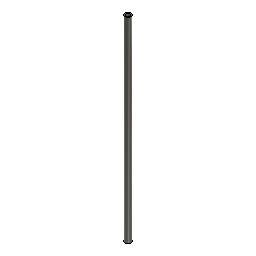
2차 예선 모델링_ADW (Autodesk Fusion 360 archive; units mm, degrees)
design "Aluminum 4mm 6mm bar"
Autodesk Fusion 360 part; units mm, degrees
sketch "Aluminum 4mm-6mm" plane through (0, 0, 0) normal (0, 0, 1) x (1, 0, 0)
  circle A0 centre (0, 0) radius 2
  circle A1 centre (0, 0) radius 3
  dimension "d1" = 4
  dimension "d2" = 6
  constraint coincident A0.centre A1.centre
  measures "d1" diameter of A0
  measures "d2" diameter of A1
extrude "Extrude1" add sketch "Aluminum 4mm-6mm" along normal blind 190 makes body 1
copy_body "Body->Comp1" bodies 1 removing the originals makes body 2 in component "190mm aluminum 4-6 bar"
extrude "Extrude2" add sketch "Aluminum 4mm-6mm" along normal blind 250 separate body makes body 3
copy_body "Body->Comp2" bodies 3 removing the originals makes body 4 in component "250mm aluminum 4-6 bar"
extrude "Extrude3" add sketch "Aluminum 4mm-6mm" along normal blind 120 separate body makes body 5
copy_body "Body->Comp3" bodies 5 removing the originals makes body 6 in component "120mm aluminum 4-6 bar"
extrude "Extrude4" add sketch "Aluminum 4mm-6mm" along normal blind 222 separate body makes body 7
copy_body "Body->Comp4" bodies 7 removing the originals makes body 8 in component "220mm aluminum 4-6 bar"
extrude "Extrude5" add sketch "Aluminum 4mm-6mm" along normal blind 30 separate body makes body 9
copy_body "Body->Comp5" bodies 9 removing the originals makes body 10 in component "30mm aluminum 4-6 bar"
component "190mm aluminum 4-6 bar" placed x (1, 0, 0) y (0, 1, 0) z (0, 0, 1) at (0, 0, 0)
component "250mm aluminum 4-6 bar" placed x (1, 0, 0) y (0, 1, 0) z (0, 0, 1) at (0, 0, 0)
component "120mm aluminum 4-6 bar" placed x (1, 0, 0) y (0, 1, 0) z (0, 0, 1) at (0, 0, 0)
component "220mm aluminum 4-6 bar" placed x (1, 0, 0) y (0, 1, 0) z (0, 0, 1) at (0, 0, 0)
component "30mm aluminum 4-6 bar" placed x (1, 0, 0) y (0, 1, 0) z (0, 0, 1) at (0, 0, 0)
equation "d13 = 180 mm + ( ( 5 + 5 + 3 + 8 ) * 2 ) * 1 mm"

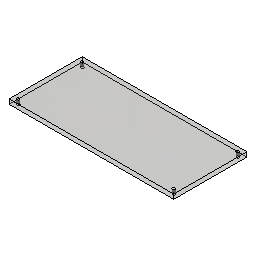
design "Simple Flat Bucket"
Autodesk Fusion 360 part; units mm, degrees
sketch "Sketch1" plane through (0, 0, 0) normal (0, 0, 1) x (1, 0, 0)
  line L0 (90, -40) -> (-90, -40)
  line L1 (-90, -40) -> (-90, 40)
  line L2 (-90, 40) -> (90, 40)
  line L3 (90, 40) -> (90, -40)
  line L4 (90, -40) -> (-90, 40) construction
  line L5 (-90, -40) -> (90, 40) construction
  line L6 (-85, -35) -> (85, 35) construction
  line L7 (85, -35) -> (-85, 35) construction
  circle A0 centre (-85, 35) radius 1.5
  circle A1 centre (-85, -35) radius 1.5
  circle A2 centre (85, 35) radius 1.5
  circle A3 centre (85, -35) radius 1.5
  dimension "d1" = 180
  dimension "d2" = 80
  dimension "d3" = 170
  dimension "d4" = 70
  dimension "d5" = 3
  dimension "d6" = 3
  dimension "d7" = 3
  dimension "d8" = 3
  constraint horizontal L0
  constraint perpendicular L0 L1
  constraint parallel L0 L2
  constraint parallel L1 L3
  constraint coincident L4 origin
  constraint coincident L5 origin
  constraint coincident L6 origin
  constraint coincident L7 origin
  constraint coincident L7.end A0.centre
  constraint coincident L6.start A1.centre
  constraint coincident L6.end A2.centre
  constraint coincident L7.start A3.centre
  measures "d1" distance of L1.end L2.end
  measures "d2" distance of L0.end L1.end
  measures "d3" distance of L6.end L7.end
  measures "d4" distance of L7.start L6.end
  measures "d5" diameter of A0
  measures "d6" diameter of A1
  measures "d7" diameter of A2
  measures "d8" diameter of A3
extrude "Extrude1" add sketch "Sketch1" along normal blind 5 makes body 1
copy_body "Body->Comp1" bodies 1 removing the originals makes body 2 in component "Simple flat bucket"
component "Simple flat bucket" placed x (1, 0, 0) y (0, 1, 0) z (0, 0, 1) at (0, 0, 0)

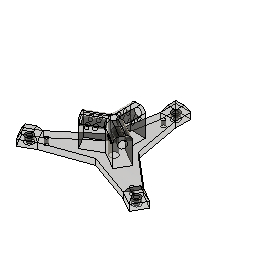
design "90mm_Center Piece 3 Cap"
Autodesk Fusion 360 part; units mm, degrees
sketch "스케치1" plane through (0, 0, 0) normal (0, 0, 1) x (1, 0, 0)
  circle A0 centre (0, 0) radius 45
  circle A1 centre (0, 0) radius 3.25
  line L0 (0, 0) -> (0, 45)
  line L1 (0, 3.25) -> (0, 7.25)
  line L2 (0, 45) -> (0, 41)
  circle A2 centre (0, 7.25) radius 1.5
  circle A3 centre (0, 41) radius 1.5
  circle A4 centre (-6.278684, -3.625) radius 1.5
  circle A5 centre (-35.507042, -20.5) radius 1.5
  circle A6 centre (6.278684, -3.625) radius 1.5
  circle A7 centre (35.507042, -20.5) radius 1.5
  line L3 (0, 45) -> (0, 57.5)
  line L4 (0, 57.5) -> (6.25, 57.5)
  line L5 (6.25, 57.5) -> (6.25, 44.563859)
  line L6 (0, 57.5) -> (-6.25, 57.5)
  line L7 (-6.25, 57.5) -> (-6.25, 44.563859)
  circle A8 centre (0, 51.25) radius 3.25
  circle A9 centre (0, 51.25) radius 1.75
  line L8 (-46.671461, -34.162659) -> (-35.468434, -27.694588)
  circle A10 centre (-44.383802, -25.625) radius 3.25
  circle A11 centre (-44.383802, -25.625) radius 1.75
  line L9 (-49.796461, -28.75) -> (-46.671461, -34.162659)
  line L10 (-49.796461, -28.75) -> (-52.921461, -23.337341)
  line L11 (-52.921461, -23.337341) -> (-41.718434, -16.869271)
  line L12 (52.921461, -23.337341) -> (41.718434, -16.869271)
  circle A12 centre (44.383802, -25.625) radius 3.25
  circle A13 centre (44.383802, -25.625) radius 1.75
  line L13 (49.796461, -28.75) -> (52.921461, -23.337341)
  line L14 (49.796461, -28.75) -> (46.671461, -34.162659)
  line L15 (46.671461, -34.162659) -> (35.468434, -27.694588)
  spline S0 degree 5 poles (35.468434, -27.694588) (34.819906, -27.317495) (33.509104, -26.546566) (31.501491, -25.340032) (28.579456, -23.675318) (23.424733, -21.747786) (16.754594, -20.597941) (9.434581, -20.121161) (3.346407, -20.006491) (0, -20) knots 0 0 0 0 0 0 0.2 0.4 0.6 0.8 1 1 1 1 1 1
  line L16 (8.439143, -20.016369) -> (-8.439143, -19.983631)
  line L17 (37.082946, -28.633365) -> (33.853922, -26.755812)
  line L18 (0, 0) -> (-0.087287, -44.999915)
  spline S1 degree 5 poles (-35.575605, -27.556783) (-34.92562, -27.182208) (-33.611836, -26.416371) (-31.599558, -25.217634) (-28.671087, -23.564268) (-23.508925, -21.656748) (-16.834376, -20.532788) (-9.512568, -20.084409) (-3.423995, -19.993358) (-0.077588, -19.99985) knots 0 0 0 0 0 0 0.2 0.4 0.6 0.8 1 1 1 1 1 1
  line L19 (-37.193747, -28.489289) -> (-33.957463, -26.624277)
  line L20 (-8.516731, -19.98348) -> (8.361555, -20.016219)
  spline S2 degree 5 poles (6.25, 44.563859) (6.247691, 43.813671) (6.235449, 42.293018) (6.194366, 39.951107) (6.213699, 36.588193) (7.121768, 31.160307) (9.461043, 24.808875) (12.708146, 18.231167) (15.652926, 12.901319) (17.320508, 10) knots 0 0 0 0 0 0 0.2 0.4 0.6 0.8 1 1 1 1 1 1
  spline S3 degree 5 poles (41.652677, -17.030986) (41.003293, -16.65537) (39.683167, -15.900518) (37.638891, -14.757203) (34.742798, -13.047755) (30.509756, -9.530952) (26.199104, -4.312603) (22.149892, 1.804079) (19.026754, 7.031413) (17.359172, 9.932731) knots 0 0 0 0 0 0 0.2 0.4 0.6 0.8 1 1 1 1 1 1
  spline S4 degree 5 poles (-41.718434, -16.869271) (-41.067597, -16.496176) (-39.744553, -15.746452) (-37.695857, -14.611075) (-34.793154, -12.912876) (-30.546501, -9.412521) (-26.215638, -4.210934) (-22.142727, 1.889994) (-18.999333, 7.105172) (-17.320508, 10) knots 0 0 0 0 0 0 0.2 0.4 0.6 0.8 1 1 1 1 1 1
  spline S5 degree 5 poles (-6.077072, 44.58777) (-6.077673, 43.837578) (-6.07133, 42.31689) (-6.039333, 39.974837) (-6.071712, 36.612024) (-7.000831, 31.1877) (-9.364728, 24.845392) (-12.637324, 18.28033) (-15.602759, 12.961946) (-17.281584, 10.067118) knots 0 0 0 0 0 0 0.2 0.4 0.6 0.8 1 1 1 1 1 1
  point P0 (0, -20)
  dimension "d1" = 90
  dimension "d2" = 6.5
  dimension "d3" = 4
  dimension "d4" = 4
  dimension "d5" = 3
  dimension "d6" = 3
  dimension "d8" = 360
  dimension "d21" = 12.5
  dimension "d22" = 6.25
  dimension "d23" = 6.5
  dimension "d24" = 3.5
  dimension "d33" = 360
  constraint coincident A0.centre A1.centre
  constraint coincident A0 L0.end
  constraint vertical L0
  constraint coincident A1 L1.start
  constraint coincident L0 L1.start
  constraint parallel L0 L1
  constraint parallel L0 L2
  constraint coincident L1.end A2.centre
  constraint coincident L2.end A3.centre
  constraint parallel L2 L3
  constraint perpendicular L3 L4
  constraint perpendicular L4 L5
  constraint symmetric L4.start L3 L6.start
  constraint symmetric L3 L4.end L6.end
  constraint midpoint L3 A8.centre
  constraint concentric A8 A9
  constraint coincident P0 S0.end
  constraint midpoint P0 L16
  constraint perpendicular L16 L18
  measures "d1" diameter of A0
  measures "d2" diameter of A1
  measures "d3" distance of L1.start L1.end
  measures "d4" distance of L0.end L2.end
  measures "d5" diameter of A2
  measures "d6" diameter of A3
  measures "d21" distance of L0.end L3.end
  measures "d22" distance of L3.end L4.end
  measures "d23" diameter of A8
  measures "d24" diameter of A9
extrude "돌출4" add sketch "스케치1" along normal blind 5 contours A0 A1 L0 L1 L2 A2 A3 S0 L16 L18 L20 | A0 L3 L4 L5 A8 | A0 L12 L13 L14 L15 | A0 A1 L0 L1 L2 A2 A3 L16 L18 S1 L20 | A0 L3 L6 L7 A8 | A0 S0 L16 L18 L20 | A0 L16 L18 S1 L20 | A0 L8 L9 L10 L11 | L0 L1 A2 | L0 L1 A2 | A4 | A6 picked at (6.734071, 29.745011) picked at (5.25, 51.10462) picked at (41.632899, -30.098943) picked at (-29.096092, -9.179545) picked at (-5.246971, 51.023662) picked at (5.130061, -28.288576) picked at (-5.231524, -28.269552) picked at (-46.882899, -21.005676) picked at (0.934562, 6.901426) picked at (-0.074521, 6.255585) picked at (-6.318535, -3.159563) picked at (6.238834, -3.159563) makes body 1
extrude "돌출5" add sketch "스케치1" along normal blind 5 draft -30 from surface at 5 contours A0 L3 L4 L5 A8 | A0 L12 L13 L14 L15 | A0 L3 L6 L7 A8 | L3 A8 A9 | L3 A8 A9 | L3 A9 | L3 A9 | A0 L8 L9 L10 L11 | A10 | A11 | A12 | A13 picked at (5.25, 51.10462) picked at (41.632899, -30.098943) picked at (-5.246971, 51.023662) picked at (-0.248404, 48.518615) picked at (2.733036, 51.012809) picked at (-0.753643, 50.736175) picked at (0.998553, 50.82811) picked at (-46.882899, -21.005676) picked at (-41.652417, -25.873404) picked at (-44.941219, -25.453059) picked at (47.115187, -25.873404) picked at (43.826384, -25.453059) bodies 1
extrude "돌출6" add sketch "스케치1" along normal blind 5 contours L3 A9 | L3 A9 | A11 | A13 picked at (-0.753643, 50.736175) picked at (0.998553, 50.82811) picked at (-44.941219, -25.453059) picked at (43.826384, -25.453059) bodies 1
copy_body "본체->구성요소2" bodies 1 removing the originals makes body 2 in component "90mm_3flapcap"
extrude "Extrude1" add 1 faces at (-27.563056, -7.985641, 5) along direction (0, 0, 1) blind 5 on bodies 2 bodies 2 in component "90mm_3flapcap"
sketch "Sketch6" plane through (0, 0, 10) normal (0, 0, 1) x (-1, 0, 0)
  line L0 (0, 0) -> (-6, 0)
  line L1 (-6, 0) -> (-6, -20)
  circle A0 centre (0, 0) radius 3.25
  line L2 (0, -3.25) -> (0, 0)
  line L3 (6, 0) -> (6, -20)
  line L4 (0, 0) -> (6, 0)
  line L5 (-6, -20) -> (6, -20)
  dimension "d36" = 6
  dimension "d37" = 20
  constraint coincident L0.start A0.centre
  constraint horizontal L0
  constraint perpendicular L0 L1
  constraint coincident A0 L2.start
  constraint perpendicular L0 L2
  constraint symmetric L0.start L2 A0.centre
  constraint symmetric L0.end L2 L3.start
  constraint symmetric L1.end L2 L3.end
  measures "d36" distance of L0.start L0.end
  measures "d37" distance of L0.end L1.end
extrude "Extrude2" add sketch "Sketch6" along normal blind 5 separate body contours L0 L1 A0 L3 L4 L5 picked at (0, -14.416667) makes body 3 in component "90mm_3flapcap"
extrude "Extrude3" add 1 faces at (0, 14.416667, 15) along direction (0, 0, 1) blind 12 on bodies 3 bodies 3 2 in component "90mm_3flapcap"
sketch "Sketch7" plane through (0, 20, 0) normal (0, 1, 0) x (-1, 0, 0)
  line L0 (-3.25, 27) -> (3.25, 27)
  line L1 (0, 27) -> (0, 24)
  line L2 (0, 24) -> (0, 21)
  circle A0 centre (0, 21) radius 3.05
  dimension "d42" = 3
  dimension "d43" = 3
  dimension "d44" = 6.1
  constraint midpoint L0 L1.start
  constraint perpendicular L0 L1
  constraint parallel L1 L2
  constraint coincident L2.end A0.centre
  measures "d42" distance of L1.start L1.end
  measures "d43" distance of L1.end L2.end
  measures "d44" diameter of A0
extrude "Extrude4" cut sketch "Sketch7" against normal blind 15 contours A0 picked at (-0.907334, 21.904758) bodies 2 3 in component "90mm_3flapcap"
fillet "Fillet1" radius 4 2 edges at (-6, 10, 27) (6, 10, 27) on bodies 3 in component "90mm_3flapcap"
sketch "Sketch8" plane through (-6, 0, 0) normal (-1, 0, 0) x (0, -1, 0)
  line L0 (-20, 10) -> (-20, 23)
  line L1 (-20, 21) -> (-5, 21)
  line L2 (-5, 21) -> (-10, 21)
  line L3 (-20, 21) -> (-15, 21)
  circle A0 centre (-15, 21) radius 1.5
  circle A1 centre (-10, 21) radius 1.5
  point P0 (-20, 21)
  point P1 (-5, 21)
  dimension "d49" = 5
  dimension "d50" = 5
  dimension "d51" = 3
  dimension "d52" = 3
  constraint coincident P0 L1.start
  constraint coincident P1 L1.end
  constraint perpendicular L0 L2
  constraint perpendicular L0 L3
  constraint coincident L3.end A0.centre
  constraint coincident L2.end A1.centre
  measures "d49" distance of P1 L2.end
  measures "d50" distance of P0 L3.end
  measures "d51" diameter of A0
  measures "d52" diameter of A1
extrude "Extrude5" cut sketch "Sketch8" against normal blind 13.303 contours L1 L3 A0 | L1 L3 A0 | L1 L2 A1 | L1 L2 A1 picked at (-15.994415, 21.074521) picked at (-14.005585, 20.925479) picked at (-10.863604, 21.498602) picked at (-10.994415, 20.925479) bodies 3 in component "90mm_3flapcap"
pattern_circular "C-Pattern1" count 3 over 360 about axis through (0, 0, 1.75) along (0, 0, 1) of bodies 3 makes body 4 at (-8.922965, -7.912292, 19.106128) makes body 5 at (11.313728, -3.771368, 19.106128) in component "90mm_3flapcap"
combine "Combine1" operation add target body 2 tool bodies 4 5 3 in component "90mm_3flapcap"
extrude "Extrude6" cut 1 faces at (-22.255559, 11.640654, 10) along direction (0, 0, -1) blind 5 on bodies 2 bodies 2 in component "90mm_3flapcap"
sketch "Sketch9" plane through (0, 0, 5) normal (0, 0, 1) x (-1, 0, 0)
  circle A0 centre (0, 0) radius 45
  line L0 (-35.468434, 27.694588) -> (-46.671461, 34.162659)
  line L1 (-41.069947, 30.928623) -> (-26.727174, 22.647819)
  arc A1 (35.468434, 27.694588) -> (-35.468434, 27.694588) centre (0, 0) ccw
  line L2 (0, 0) -> (0, 45)
  line L3 (-35.468434, 27.694588) -> (0, 15)
  line L4 (35.468434, 27.694588) -> (0, 15)
  line L5 (-6.25, -44.563859) -> (-12.990381, -7.5)
  line L6 (-41.718434, 16.869271) -> (-12.990381, -7.5)
  line L7 (41.718434, 16.869271) -> (12.990381, -7.5)
  line L8 (6.25, -44.563859) -> (12.990381, -7.5)
  line L9 (0, 0) -> (0, 15)
  dimension "d60" = 360
  dimension "d63" = 15
  constraint coincident A0.centre A1.centre
  constraint parallel L0 L1
  constraint midpoint A1 L2.end
  constraint coincident L2 L3.end
  constraint symmetric L2 L3.end L4.end
  constraint parallel L2 L9
  constraint coincident L3.end L4.end
  measures "d63" distance of A0.centre L3.end
extrude "Extrude7" cut sketch "Sketch9" against normal blind 25 contours A0 L7 L8 | A0 A1 L2 L4 | A0 L5 L6 | A0 A1 L2 L3 picked at (30.575697, -16.872457) picked at (1.939961, 34.874023) picked at (-30.247561, -17.463438) picked at (-1.939961, 34.874023) bodies 2 in component "90mm_3flapcap"
component "90mm_3flapcap" placed x (1, 0, 0) y (0, 1, 0) z (0, 0, 1) at (0, 0, 0)
equation "d21 = 6.5 mm + ( 3 * 2 ) * 1 mm"
equation "d22 = ( 6.5 / 2 ) * 1 mm + 3 mm"

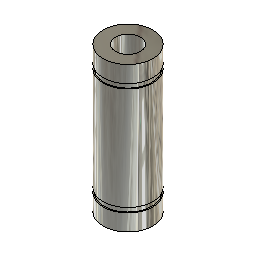
design "LM6L"
Autodesk Fusion 360 part; units mm, degrees
sketch "Sketch1" plane through (0, 0, 0) normal (0, 0, 1) x (1, 0, 0)
  circle A0 centre (0, 0) radius 6
  circle A1 centre (0, 0) radius 3
  dimension "d1" = 12
  dimension "d2" = 6
  constraint coincident A0.centre A1.centre
  constraint concentric A0 A1
  measures "d1" diameter of A0
  measures "d2" diameter of A1
extrude "Extrude1" add sketch "Sketch1" along normal blind 35 makes body 1
sketch "Sketch2" plane through (0, 0, 35) normal (0, 0, 1) x (-1, 0, 0)
  circle A0 centre (0, 0) radius 5.75
  circle A1 centre (0, 0) radius 6
  dimension "d5" = 11.5
  dimension "d6" = 12
  constraint coincident A0.centre A1.centre
  measures "d5" diameter of A0
  measures "d6" diameter of A1
extrude "Extrude2" add sketch "Sketch2" against normal blind 1.1 from surface at -4 separate body makes body 2
ref_plane "WorkPlane1" through (0, 0, 17.5) normal (0, 0, -1) x (-1, 0, 0)
mirror "Mirror1" about plane through (0, 0, 17.5) normal (0, 0, -1) of bodies 2 makes body 3
combine "Combine1" operation cut target body 1 tool bodies 2 3
copy_body "Body->Comp1" bodies 1 removing the originals makes body 4 in component "LM6L"
component "LM6L" placed x (1, 0, 0) y (0, 1, 0) z (0, 0, 1) at (0, 0, 0)
equation "d7 = ( -( 35 - 27 ) / 2 ) * 1 mm"
named bodies: "LM6L"

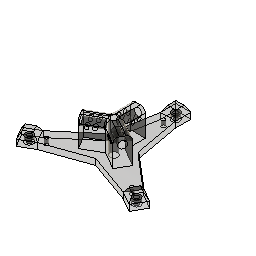
design "90mm_Center Piece 3 Cap"
Autodesk Fusion 360 part; units mm, degrees
sketch "스케치1" plane through (0, 0, 0) normal (0, 0, 1) x (1, 0, 0)
  circle A0 centre (0, 0) radius 45
  circle A1 centre (0, 0) radius 3.25
  line L0 (0, 0) -> (0, 45)
  line L1 (0, 3.25) -> (0, 7.25)
  line L2 (0, 45) -> (0, 41)
  circle A2 centre (0, 7.25) radius 1.5
  circle A3 centre (0, 41) radius 1.5
  circle A4 centre (-6.278684, -3.625) radius 1.5
  circle A5 centre (-35.507042, -20.5) radius 1.5
  circle A6 centre (6.278684, -3.625) radius 1.5
  circle A7 centre (35.507042, -20.5) radius 1.5
  line L3 (0, 45) -> (0, 57.5)
  line L4 (0, 57.5) -> (6.25, 57.5)
  line L5 (6.25, 57.5) -> (6.25, 44.563859)
  line L6 (0, 57.5) -> (-6.25, 57.5)
  line L7 (-6.25, 57.5) -> (-6.25, 44.563859)
  circle A8 centre (0, 51.25) radius 3.25
  circle A9 centre (0, 51.25) radius 1.75
  line L8 (-46.671461, -34.162659) -> (-35.468434, -27.694588)
  circle A10 centre (-44.383802, -25.625) radius 3.25
  circle A11 centre (-44.383802, -25.625) radius 1.75
  line L9 (-49.796461, -28.75) -> (-46.671461, -34.162659)
  line L10 (-49.796461, -28.75) -> (-52.921461, -23.337341)
  line L11 (-52.921461, -23.337341) -> (-41.718434, -16.869271)
  line L12 (52.921461, -23.337341) -> (41.718434, -16.869271)
  circle A12 centre (44.383802, -25.625) radius 3.25
  circle A13 centre (44.383802, -25.625) radius 1.75
  line L13 (49.796461, -28.75) -> (52.921461, -23.337341)
  line L14 (49.796461, -28.75) -> (46.671461, -34.162659)
  line L15 (46.671461, -34.162659) -> (35.468434, -27.694588)
  spline S0 degree 5 poles (35.468434, -27.694588) (34.819906, -27.317495) (33.509104, -26.546566) (31.501491, -25.340032) (28.579456, -23.675318) (23.424733, -21.747786) (16.754594, -20.597941) (9.434581, -20.121161) (3.346407, -20.006491) (0, -20) knots 0 0 0 0 0 0 0.2 0.4 0.6 0.8 1 1 1 1 1 1
  line L16 (8.439143, -20.016369) -> (-8.439143, -19.983631)
  line L17 (37.082946, -28.633365) -> (33.853922, -26.755812)
  line L18 (0, 0) -> (-0.087287, -44.999915)
  spline S1 degree 5 poles (-35.575605, -27.556783) (-34.92562, -27.182208) (-33.611836, -26.416371) (-31.599558, -25.217634) (-28.671087, -23.564268) (-23.508925, -21.656748) (-16.834376, -20.532788) (-9.512568, -20.084409) (-3.423995, -19.993358) (-0.077588, -19.99985) knots 0 0 0 0 0 0 0.2 0.4 0.6 0.8 1 1 1 1 1 1
  line L19 (-37.193747, -28.489289) -> (-33.957463, -26.624277)
  line L20 (-8.516731, -19.98348) -> (8.361555, -20.016219)
  spline S2 degree 5 poles (6.25, 44.563859) (6.247691, 43.813671) (6.235449, 42.293018) (6.194366, 39.951107) (6.213699, 36.588193) (7.121768, 31.160307) (9.461043, 24.808875) (12.708146, 18.231167) (15.652926, 12.901319) (17.320508, 10) knots 0 0 0 0 0 0 0.2 0.4 0.6 0.8 1 1 1 1 1 1
  spline S3 degree 5 poles (41.652677, -17.030986) (41.003293, -16.65537) (39.683167, -15.900518) (37.638891, -14.757203) (34.742798, -13.047755) (30.509756, -9.530952) (26.199104, -4.312603) (22.149892, 1.804079) (19.026754, 7.031413) (17.359172, 9.932731) knots 0 0 0 0 0 0 0.2 0.4 0.6 0.8 1 1 1 1 1 1
  spline S4 degree 5 poles (-41.718434, -16.869271) (-41.067597, -16.496176) (-39.744553, -15.746452) (-37.695857, -14.611075) (-34.793154, -12.912876) (-30.546501, -9.412521) (-26.215638, -4.210934) (-22.142727, 1.889994) (-18.999333, 7.105172) (-17.320508, 10) knots 0 0 0 0 0 0 0.2 0.4 0.6 0.8 1 1 1 1 1 1
  spline S5 degree 5 poles (-6.077072, 44.58777) (-6.077673, 43.837578) (-6.07133, 42.31689) (-6.039333, 39.974837) (-6.071712, 36.612024) (-7.000831, 31.1877) (-9.364728, 24.845392) (-12.637324, 18.28033) (-15.602759, 12.961946) (-17.281584, 10.067118) knots 0 0 0 0 0 0 0.2 0.4 0.6 0.8 1 1 1 1 1 1
  point P0 (0, -20)
  dimension "d1" = 90
  dimension "d2" = 6.5
  dimension "d3" = 4
  dimension "d4" = 4
  dimension "d5" = 3
  dimension "d6" = 3
  dimension "d8" = 360
  dimension "d21" = 12.5
  dimension "d22" = 6.25
  dimension "d23" = 6.5
  dimension "d24" = 3.5
  dimension "d33" = 360
  constraint coincident A0.centre A1.centre
  constraint coincident A0 L0.end
  constraint vertical L0
  constraint coincident A1 L1.start
  constraint coincident L0 L1.start
  constraint parallel L0 L1
  constraint parallel L0 L2
  constraint coincident L1.end A2.centre
  constraint coincident L2.end A3.centre
  constraint parallel L2 L3
  constraint perpendicular L3 L4
  constraint perpendicular L4 L5
  constraint symmetric L4.start L3 L6.start
  constraint symmetric L3 L4.end L6.end
  constraint midpoint L3 A8.centre
  constraint concentric A8 A9
  constraint coincident P0 S0.end
  constraint midpoint P0 L16
  constraint perpendicular L16 L18
  measures "d1" diameter of A0
  measures "d2" diameter of A1
  measures "d3" distance of L1.start L1.end
  measures "d4" distance of L0.end L2.end
  measures "d5" diameter of A2
  measures "d6" diameter of A3
  measures "d21" distance of L0.end L3.end
  measures "d22" distance of L3.end L4.end
  measures "d23" diameter of A8
  measures "d24" diameter of A9
extrude "돌출4" add sketch "스케치1" along normal blind 5 contours A0 A1 L0 L1 L2 A2 A3 S0 L16 L18 L20 | A0 L3 L4 L5 A8 | A0 L12 L13 L14 L15 | A0 A1 L0 L1 L2 A2 A3 L16 L18 S1 L20 | A0 L3 L6 L7 A8 | A0 S0 L16 L18 L20 | A0 L16 L18 S1 L20 | A0 L8 L9 L10 L11 | L0 L1 A2 | L0 L1 A2 | A4 | A6 picked at (6.734071, 29.745011) picked at (5.25, 51.10462) picked at (41.632899, -30.098943) picked at (-29.096092, -9.179545) picked at (-5.246971, 51.023662) picked at (5.130061, -28.288576) picked at (-5.231524, -28.269552) picked at (-46.882899, -21.005676) picked at (0.934562, 6.901426) picked at (-0.074521, 6.255585) picked at (-6.318535, -3.159563) picked at (6.238834, -3.159563) makes body 1
extrude "돌출5" add sketch "스케치1" along normal blind 5 draft -30 from surface at 5 contours A0 L3 L4 L5 A8 | A0 L12 L13 L14 L15 | A0 L3 L6 L7 A8 | L3 A8 A9 | L3 A8 A9 | L3 A9 | L3 A9 | A0 L8 L9 L10 L11 | A10 | A11 | A12 | A13 picked at (5.25, 51.10462) picked at (41.632899, -30.098943) picked at (-5.246971, 51.023662) picked at (-0.248404, 48.518615) picked at (2.733036, 51.012809) picked at (-0.753643, 50.736175) picked at (0.998553, 50.82811) picked at (-46.882899, -21.005676) picked at (-41.652417, -25.873404) picked at (-44.941219, -25.453059) picked at (47.115187, -25.873404) picked at (43.826384, -25.453059) bodies 1
extrude "돌출6" add sketch "스케치1" along normal blind 5 contours L3 A9 | L3 A9 | A11 | A13 picked at (-0.753643, 50.736175) picked at (0.998553, 50.82811) picked at (-44.941219, -25.453059) picked at (43.826384, -25.453059) bodies 1
copy_body "본체->구성요소2" bodies 1 removing the originals makes body 2 in component "90mm_3flapcap"
extrude "Extrude1" add 1 faces at (-27.563056, -7.985641, 5) along direction (0, 0, 1) blind 5 on bodies 2 bodies 2 in component "90mm_3flapcap"
sketch "Sketch6" plane through (0, 0, 10) normal (0, 0, 1) x (-1, 0, 0)
  line L0 (0, 0) -> (-6, 0)
  line L1 (-6, 0) -> (-6, -20)
  circle A0 centre (0, 0) radius 3.25
  line L2 (0, -3.25) -> (0, 0)
  line L3 (6, 0) -> (6, -20)
  line L4 (0, 0) -> (6, 0)
  line L5 (-6, -20) -> (6, -20)
  dimension "d36" = 6
  dimension "d37" = 20
  constraint coincident L0.start A0.centre
  constraint horizontal L0
  constraint perpendicular L0 L1
  constraint coincident A0 L2.start
  constraint perpendicular L0 L2
  constraint symmetric L0.start L2 A0.centre
  constraint symmetric L0.end L2 L3.start
  constraint symmetric L1.end L2 L3.end
  measures "d36" distance of L0.start L0.end
  measures "d37" distance of L0.end L1.end
extrude "Extrude2" add sketch "Sketch6" along normal blind 5 separate body contours L0 L1 A0 L3 L4 L5 picked at (0, -14.416667) makes body 3 in component "90mm_3flapcap"
extrude "Extrude3" add 1 faces at (0, 14.416667, 15) along direction (0, 0, 1) blind 12 on bodies 3 bodies 3 2 in component "90mm_3flapcap"
sketch "Sketch7" plane through (0, 20, 0) normal (0, 1, 0) x (-1, 0, 0)
  line L0 (-3.25, 27) -> (3.25, 27)
  line L1 (0, 27) -> (0, 24)
  line L2 (0, 24) -> (0, 21)
  circle A0 centre (0, 21) radius 3.05
  dimension "d42" = 3
  dimension "d43" = 3
  dimension "d44" = 6.1
  constraint midpoint L0 L1.start
  constraint perpendicular L0 L1
  constraint parallel L1 L2
  constraint coincident L2.end A0.centre
  measures "d42" distance of L1.start L1.end
  measures "d43" distance of L1.end L2.end
  measures "d44" diameter of A0
extrude "Extrude4" cut sketch "Sketch7" against normal blind 15 contours A0 picked at (-0.907334, 21.904758) bodies 2 3 in component "90mm_3flapcap"
fillet "Fillet1" radius 4 2 edges at (-6, 10, 27) (6, 10, 27) on bodies 3 in component "90mm_3flapcap"
sketch "Sketch8" plane through (-6, 0, 0) normal (-1, 0, 0) x (0, -1, 0)
  line L0 (-20, 10) -> (-20, 23)
  line L1 (-20, 21) -> (-5, 21)
  line L2 (-5, 21) -> (-10, 21)
  line L3 (-20, 21) -> (-15, 21)
  circle A0 centre (-15, 21) radius 1.5
  circle A1 centre (-10, 21) radius 1.5
  point P0 (-20, 21)
  point P1 (-5, 21)
  dimension "d49" = 5
  dimension "d50" = 5
  dimension "d51" = 3
  dimension "d52" = 3
  constraint coincident P0 L1.start
  constraint coincident P1 L1.end
  constraint perpendicular L0 L2
  constraint perpendicular L0 L3
  constraint coincident L3.end A0.centre
  constraint coincident L2.end A1.centre
  measures "d49" distance of P1 L2.end
  measures "d50" distance of P0 L3.end
  measures "d51" diameter of A0
  measures "d52" diameter of A1
extrude "Extrude5" cut sketch "Sketch8" against normal blind 13.303 contours L1 L3 A0 | L1 L3 A0 | L1 L2 A1 | L1 L2 A1 picked at (-15.994415, 21.074521) picked at (-14.005585, 20.925479) picked at (-10.863604, 21.498602) picked at (-10.994415, 20.925479) bodies 3 in component "90mm_3flapcap"
pattern_circular "C-Pattern1" count 3 over 360 about axis through (0, 0, 1.75) along (0, 0, 1) of bodies 3 makes body 4 at (-8.922965, -7.912292, 19.106128) makes body 5 at (11.313728, -3.771368, 19.106128) in component "90mm_3flapcap"
combine "Combine1" operation add target body 2 tool bodies 4 5 3 in component "90mm_3flapcap"
extrude "Extrude6" cut 1 faces at (-22.255559, 11.640654, 10) along direction (0, 0, -1) blind 5 on bodies 2 bodies 2 in component "90mm_3flapcap"
sketch "Sketch9" plane through (0, 0, 5) normal (0, 0, 1) x (-1, 0, 0)
  circle A0 centre (0, 0) radius 45
  line L0 (-35.468434, 27.694588) -> (-46.671461, 34.162659)
  line L1 (-41.069947, 30.928623) -> (-26.727174, 22.647819)
  arc A1 (35.468434, 27.694588) -> (-35.468434, 27.694588) centre (0, 0) ccw
  line L2 (0, 0) -> (0, 45)
  line L3 (-35.468434, 27.694588) -> (0, 15)
  line L4 (35.468434, 27.694588) -> (0, 15)
  line L5 (-6.25, -44.563859) -> (-12.990381, -7.5)
  line L6 (-41.718434, 16.869271) -> (-12.990381, -7.5)
  line L7 (41.718434, 16.869271) -> (12.990381, -7.5)
  line L8 (6.25, -44.563859) -> (12.990381, -7.5)
  line L9 (0, 0) -> (0, 15)
  dimension "d60" = 360
  dimension "d63" = 15
  constraint coincident A0.centre A1.centre
  constraint parallel L0 L1
  constraint midpoint A1 L2.end
  constraint coincident L2 L3.end
  constraint symmetric L2 L3.end L4.end
  constraint parallel L2 L9
  constraint coincident L3.end L4.end
  measures "d63" distance of A0.centre L3.end
extrude "Extrude7" cut sketch "Sketch9" against normal blind 25 contours A0 L7 L8 | A0 A1 L2 L4 | A0 L5 L6 | A0 A1 L2 L3 picked at (30.575697, -16.872457) picked at (1.939961, 34.874023) picked at (-30.247561, -17.463438) picked at (-1.939961, 34.874023) bodies 2 in component "90mm_3flapcap"
component "90mm_3flapcap" placed x (1, 0, 0) y (0, 1, 0) z (0, 0, 1) at (0, 0, 0)
equation "d21 = 6.5 mm + ( 3 * 2 ) * 1 mm"
equation "d22 = ( 6.5 / 2 ) * 1 mm + 3 mm"

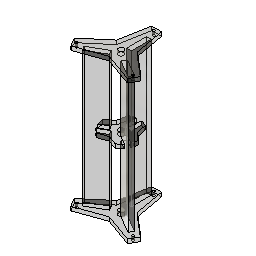
design "Center 90mm_Center Piece_3 flaps" references "90mm_Center Piece 3 Cap"
Autodesk Fusion 360 part; units mm, degrees
sketch "스케치1" plane through (0, 0, 0) normal (0, 0, 1) x (1, 0, 0)
  circle A0 centre (0, 0) radius 45
  circle A1 centre (0, 0) radius 3.25
  line L0 (0, 0) -> (0, 45)
  line L1 (0, 3.25) -> (0, 7.25)
  line L2 (0, 45) -> (0, 41)
  circle A2 centre (0, 7.25) radius 1.5
  circle A3 centre (0, 41) radius 1.5
  circle A4 centre (-6.2787, -3.625) radius 1.5
  circle A5 centre (-35.507, -20.5) radius 1.5
  circle A6 centre (6.2787, -3.625) radius 1.5
  circle A7 centre (35.507, -20.5) radius 1.5
  dimension "d1" = 90
  dimension "d2" = 6.5
  dimension "d3" = 4
  dimension "d4" = 4
  dimension "d5" = 3
  dimension "d6" = 3
  dimension "d22" = 360
  constraint coincident A0.centre A1.centre
  constraint coincident A0 L0.end
  constraint vertical L0
  constraint coincident A1 L1.start
  constraint coincident L0 L1.start
  constraint parallel L0 L1
  constraint parallel L0 L2
  constraint coincident L1.end A2.centre
  constraint coincident L2.end A3.centre
  measures "d1" diameter of A0
  measures "d2" diameter of A1
  measures "d3" distance of L1.start L1.end
  measures "d4" distance of L0.end L2.end
  measures "d5" diameter of A2
  measures "d6" diameter of A3
extrude "돌출1" add sketch "스케치1" along normal blind 5 contours A0 | L0 L1 A2 | L0 L1 A2 | A4 | A6 makes body 1
sketch "스케치4" plane through (0, 0, 5) normal (0, 0, 1) x (-1, 0, 0)
  line L0 (0, 0) -> (11.25, 19.4856) construction
  line L1 (0, 0) -> (11.25, 19.4856) construction
  line L2 (0, 0) -> (17.5, 30.3109) construction
  line L3 (8.6603, 5) -> (30.3109, 17.5)
  dimension "d25" = 35
  dimension "d27" = 10
  constraint coincident L0.start L1.start
  measures "d25" distance of L0.start L3.end
  measures "d27" distance of L0.start L3.start
surface "돌출2" add extruded along (0, 0, 1) between 0 and 170 path "스케치4" along L3 separate body makes body 2
thicken "두껍게 하기1" add thickness 3 on both sides surfaces 2 separate body makes body 3
copy_body "CopyPasteBodies1" bodies 1 makes body 4
move_body "이동1" bodies 4 to x (1, 0, 0) y (0, 1, 0) z (0, 0, 1) at (0, 0, 175)
pattern_circular "C-패턴1" count 3 over 360 about axis through (0, 0, 1.75) along (0, 0, 1) of bodies 3 2 makes body 5 at (15.8771, -9.1667, 61.6667) makes body 6 at (0, 18.3333, 61.6667) makes body 7 at (17.3771, -6.5686, 61.6667) makes body 8 at (-3, 18.3333, 61.6667)
sketch "스케치5" plane through (0, 0, 180) normal (0, 0, 1) x (-1, 0, 0)
  circle A0 centre (0, 0) radius 22.5
  circle A1 centre (0, 0) radius 3.25
  constraint coincident A0.centre A1.centre
extrude "돌출3" add sketch "스케치5" against normal blind 5 from surface at -87.5 separate body makes body 9
delete_body "RemoveBody11" bodies 5
delete_body "RemoveBody12" bodies 6
delete_body "RemoveBody15" bodies 2
combine "Combine2" operation add target body 9 tool bodies 4 3 7 8 1
copy_body "본체->구성요소1" bodies 9 removing the originals makes body 10 in component "90mm_Center Piece_3flaps"
derive "Sketch9" from "90mm_Center Piece 3 Cap v5"
sketch "sketch 2727" plane through (0, 0, 5) normal (0, 0, 1) x (-1, 0, 0)
  circle A0 centre (0, 0) radius 45
  line L0 (-35.4684, 27.6946) -> (-46.6715, 34.1627)
  line L1 (-41.0699, 30.9286) -> (-26.7272, 22.6478)
  arc A1 (35.4684, 27.6946) -> (-35.4684, 27.6946) centre (0, 0) ccw
  line L2 (0, 0) -> (0, 45)
  line L3 (-35.4684, 27.6946) -> (0, 15)
  line L4 (35.4684, 27.6946) -> (0, 15)
  line L5 (-6.25, -44.5639) -> (-12.9904, -7.5)
  line L6 (-41.7184, 16.8693) -> (-12.9904, -7.5)
  line L7 (41.7184, 16.8693) -> (12.9904, -7.5)
  line L8 (6.25, -44.5639) -> (12.9904, -7.5)
  line L9 (0, 0) -> (0, 15)
extrude "Extrude1" cut sketch "sketch 2727" along normal blind 175 and the other way blind 5 contours A0 L7 L8 | A0 A1 L2 L4 | A0 L5 L6 | A0 A1 L2 L3 bodies 10 in component "90mm_Center Piece_3flaps"
component "90mm_Center Piece_3flaps" placed x (1, 0, 0) y (0, 1, 0) z (0, 0, 1) at (0, 0, 0)
equation "d18 = ( -( 180 - 5 ) / 2 ) * 1 mm"

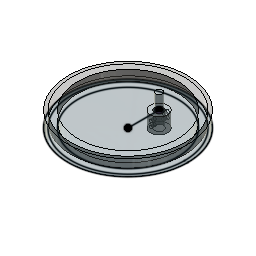
design "Simple Cam, 30mm"
Autodesk Fusion 360 part; units mm, degrees
sketch "Sketch1" plane through (0, 0, 0) normal (0, 0, 1) x (1, 0, 0)
  line L0 (0, 0) -> (0, -30)
  circle A0 centre (0, -30) radius 54.5
  circle A1 centre (0, -30) radius 48
  circle A2 centre (0, 0) radius 3.25
  circle A3 centre (0, -30) radius 57.5
  dimension "d1" = 30
  dimension "d2" = 109
  dimension "d3" = 96
  dimension "d4" = 6.5
  dimension "d5" = 115
  constraint coincident L0.start A2.centre
  constraint vertical L0
  constraint coincident L0.end A0.centre
  constraint concentric A0 A1
  constraint concentric A1 A3
  measures "d1" distance of L0.start L0.end
  measures "d2" diameter of A0
  measures "d3" diameter of A1
  measures "d4" diameter of A2
  measures "d5" diameter of A3
extrude "Extrude1" add sketch "Sketch1" along normal blind 5 contours A0 | A1 | A3 makes body 1
extrude "Extrude2" add sketch "Sketch1" along normal blind 10 from surface at 5 bodies 1
sketch "Sketch2" plane through (0, 0, 0) normal (0, 0, 1) x (1, 0, 0)
  circle A0 centre (0, 0) radius 8.25
  circle A1 centre (0, 0) radius 4.29
  dimension "d11" = 16.5
  constraint coincident A0.centre A1.centre
  constraint concentric A0 A1
  measures "d11" diameter of A0
extrude "Extrude3" add sketch "Sketch2" against normal blind 15 bodies 1
sketch "Sketch4" plane through (0, 0, 0) normal (0, 1, 0) x (1, 0, 0)
  line L0 (-4.29, 15) -> (4.29, 15)
  line L1 (0, 0) -> (0, 15)
  line L2 (-8.25, 0) -> (8.25, 0)
  line L3 (0, 0) -> (0, 5)
  line L4 (0, 15) -> (0, 14)
  line L5 (0, 15) -> (0, 10)
  circle A0 centre (0, 5) radius 1.5
  circle A1 centre (0, 10) radius 1.5
  dimension "d14" = 5
  dimension "d15" = 5
  dimension "d16" = 3
  dimension "d17" = 3
  constraint coincident L1.start L3.start
  constraint midpoint L0 L1.end
  constraint perpendicular L2 L3
  constraint coincident L1 L4.end
  constraint perpendicular L0 L4
  constraint coincident L1 L5.end
  constraint coincident L3.end A0.centre
  constraint coincident L5.end A1.centre
  measures "d14" distance of L1.start L3.end
  measures "d15" distance of L1.end L5.end
  measures "d16" diameter of A0
  measures "d17" diameter of A1
extrude "Extrude4" cut sketch "Sketch4" along normal mid plane 20 bodies 1
copy_body "Body->Comp1" bodies 1 removing the originals makes body 2 in component "Simple Cam, 30mm "
component "Simple Cam, 30mm " placed x (1, 0, 0) y (0, 1, 0) z (0, 0, 1) at (0, 0, 0)
equation "d1 = ( 102.5 / 2 ) * 1 mm - 21.25 mm"
equation "d2 = 102.5 mm + 6.5 mm"
equation "d3 = 102.5 mm - 6.5 mm"
equation "d5 = 102.5 mm + 6.5 mm + ( 3 * 2 ) * 1 mm"
equation "d11 = 6.5 mm + ( 5 * 2 ) * 1 mm"

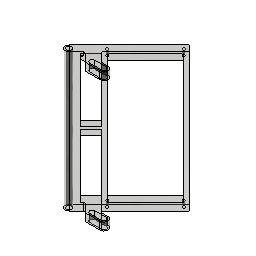
design "Cam version flap, L = 30mm"
Autodesk Fusion 360 part; units mm, degrees
sketch "Sketch1" plane through (0, 0, 0) normal (0, 0, 1) x (1, 0, 0)
  circle A0 centre (0, 0) radius 3.25
  line L0 (0, 0) -> (0, -3.25)
  line L1 (0, -3.25) -> (0, -5.25)
  line L2 (0, -6.25) -> (0, -28.75)
  circle A1 centre (0, -28.75) radius 22.5
  circle A2 centre (0, 0) radius 5.25
  line L3 (0, -5.25) -> (5.25, -5.25)
  line L4 (0, 0) -> (0, 110)
  line L5 (5.25, 5.25) -> (5.25, 110)
  line L6 (0, 110) -> (5.25, 110)
  line L7 (0, 110) -> (-5.25, 110)
  line L8 (-5.25, 110) -> (-5.25, 0)
  line L9 (5.25, 5.25) -> (5.25, 0)
  dimension "d1" = 6.5
  dimension "d2" = 2
  dimension "d3" = 1
  dimension "d4" = 22.5
  dimension "d5" = 5.25
  dimension "d9" = 110
  dimension "d10" = 104.75
  dimension "d11" = 5.25
  constraint coincident A0.centre L0.start
  constraint coincident A0 L0.end
  constraint vertical L0
  constraint parallel L0 L1
  constraint coincident L2.end A1.centre
  constraint coincident L2.start A1
  constraint coincident L1.end A2
  constraint perpendicular L1 L3
  constraint parallel L0 L4
  constraint perpendicular L4 L7
  constraint coincident A2 L8.end
  constraint tangent A2 L8
  constraint coincident A2 L9.end
  constraint tangent A2 L9
  constraint parallel L5 L9
  measures "d1" diameter of A0
  measures "d2" distance of L0.end L1.end
  measures "d3" distance of L1.end L2.start
  measures "d4" distance of L2.start L2.end
  measures "d5" distance of L1.end L3.end
  measures "d9" distance of A0.centre L4.end
  measures "d10" distance of L5.start L5.end
  measures "d11" distance of L4.end L7.end
extrude "Extrude1" add sketch "Sketch1" along normal blind 179 contours A0 L1 A2 L4 | A0 L1 A2 L4 | A2 L4 L5 L6 L9 | A2 L4 L7 L8 makes body 1
sketch "Sketch2" plane through (-5.25, 0, 0) normal (-1, 0, 0) x (0, -1, 0)
  line L0 (-110, 0) -> (-110, 179)
  line L1 (-110, 89.5) -> (-5.25, 89.5)
  line L2 (-110, 89.5) -> (-70, 89.5)
  line L3 (-35, 169.5) -> (-105, 169.5)
  line L4 (-105, 169.5) -> (-105, 9.5)
  line L5 (-105, 9.5) -> (-35, 9.5)
  line L6 (-35, 9.5) -> (-35, 169.5)
  line L7 (-35, 169.5) -> (-105, 9.5) construction
  line L8 (-105, 169.5) -> (-35, 9.5) construction
  line L9 (-105, 174.5) -> (-35, 174.5)
  line L10 (-35, 174.5) -> (-35, 4.5)
  line L11 (-35, 4.5) -> (-105, 4.5)
  line L12 (-105, 4.5) -> (-105, 174.5)
  line L13 (-105, 174.5) -> (-35, 4.5) construction
  line L14 (-35, 174.5) -> (-105, 4.5) construction
  circle A0 centre (-105, 174.5) radius 1.5
  circle A1 centre (-35, 174.5) radius 1.5
  circle A2 centre (-105, 4.5) radius 1.5
  circle A3 centre (-35, 4.5) radius 1.5
  point P0 (-70, 89.5)
  point P1 (-70, 89.5)
  dimension "d14" = 40
  dimension "d15" = 70
  dimension "d16" = 160
  dimension "d23" = 70
  dimension "d24" = 170
  dimension "d25" = 3
  dimension "d26" = 3
  dimension "d27" = 3
  dimension "d28" = 3
  constraint midpoint L0 L1.start
  constraint perpendicular L0 L2
  constraint horizontal L3
  constraint perpendicular L3 L4
  constraint parallel L3 L5
  constraint parallel L4 L6
  constraint coincident L7 P1
  constraint coincident L8 P1
  constraint coincident P1 P0
  constraint horizontal L9
  constraint perpendicular L9 L10
  constraint parallel L9 L11
  constraint parallel L10 L12
  constraint coincident L13 P1
  constraint coincident L14 P1
  constraint coincident L9.start L12.end
  constraint coincident L9.end L10.start
  constraint coincident L11.end L12.start
  constraint coincident L10.end L11.start
  measures "d14" distance of L1.start P1
  measures "d15" distance of L4.end L5.end
  measures "d16" distance of L3.end L4.end
  measures "d23" distance of L10.end L11.end
  measures "d24" distance of L9.end L10.end
  measures "d25" diameter of A0
  measures "d26" diameter of A1
  measures "d27" diameter of A2
  measures "d28" diameter of A3
extrude "Extrude2" cut sketch "Sketch2" against normal blind 10.5 contours L1 L2 L3 L4 L6 L10 L12 | L1 L2 L4 L5 L6 L10 L12 | L9 L12 A0 | L9 L12 A0 | L11 L12 A2 | L11 L12 A2 | L9 L10 A1 | L9 L10 A1 | L10 L11 A3 | L10 L11 A3 bodies 1
sketch "Sketch3" plane through (-5.25, 0, 0) normal (-1, 0, 0) x (0, -1, 0)
  line L0 (-35, 9.5) -> (-35, 169.5)
  line L1 (-35, 89.5) -> (-5.25, 89.5)
  line L2 (-110, 0) -> (0, 0)
  line L3 (-20.125, 89.5) -> (-20.125, 0)
  line L4 (-110, 179) -> (0, 179)
  line L5 (-20.125, 89.5) -> (-20.125, 179)
  line L6 (-20.125, 89.5) -> (-20.125, 0)
  line L7 (-10.25, 84.5) -> (-30, 84.5)
  line L8 (-30, 84.5) -> (-30, 5)
  line L9 (-30, 5) -> (-10.25, 5)
  line L10 (-10.25, 5) -> (-10.25, 84.5)
  line L11 (-10.25, 84.5) -> (-30, 5) construction
  line L12 (-30, 84.5) -> (-10.25, 5) construction
  line L13 (-10.25, 94.5) -> (-30, 94.5)
  line L14 (-30, 94.5) -> (-30, 174)
  line L15 (-10.25, 174) -> (-10.25, 94.5)
  line L16 (-30, 174) -> (-10.25, 174)
  point P0 (-20.125, 44.75)
  point P1 (-20.125, 44.75)
  dimension "d19" = 19.75
  dimension "d20" = 79.5
  constraint midpoint L0 L1.start
  constraint midpoint L1 L3.start
  constraint coincident L2 L3.end
  constraint perpendicular L1 L3
  constraint coincident L4 L5.end
  constraint perpendicular L1 L5
  constraint midpoint L6 P1
  constraint horizontal L7
  constraint perpendicular L7 L8
  constraint parallel L7 L9
  constraint parallel L8 L10
  constraint coincident L11 P1
  constraint coincident L12 P1
  constraint coincident P1 P0
  constraint symmetric L1 L7.start L13.start
  constraint symmetric L1 L7.end L13.end
  constraint symmetric L1 L8.end L14.end
  constraint symmetric L1 L9.end L15.start
  measures "d19" distance of L8.end L9.end
  measures "d20" distance of L7.end L8.end
extrude "Extrude3" cut sketch "Sketch3" against normal blind 25 bodies 1
sketch "Sketch4" plane through (-5.25, 0, 0) normal (-1, 0, 0) x (0, -1, 0)
copy_body "Body->Comp1" bodies 1 removing the originals makes body 2 in component "Cam version flap L = 30mm"
move_body "Move1" bodies 2 to x (0.707107, -0.707107, 0) y (0.707107, 0.707107, 0) z (0, 0, 1) at (0, 0, 0) in component "Cam version flap L = 30mm"
sketch "Sketch5" plane through (0, 0, 0) normal (0, 0, 1) x (1, 0, 0)
  line L0 (0, 0) -> (30, 0)
  line L1 (0, 0) -> (45, 0)
  line L2 (0, -5.25) -> (45, -5.25)
  arc A0 (45, -5.25) -> (45, 5.25) centre (45, 0) ccw
  line L3 (45, 5.25) -> (0, 5.25)
  arc A1 (0, 5.25) -> (0, -5.25) centre (0, 0) ccw
  line L4 (0, 0) -> (45, 0) construction
  line L5 (30, -3.25) -> (45, -3.25)
  arc A2 (45, -3.25) -> (45, 3.25) centre (45, 0) ccw
  line L6 (45, 3.25) -> (30, 3.25)
  arc A3 (30, 3.25) -> (30, -3.25) centre (30, 0) ccw
  line L7 (30, 0) -> (45, 0) construction
  circle A4 centre (0, 0) radius 3.25
  line L8 (3.5355, 10.9602) -> (10.9602, 3.5355)
  line L9 (0, 0) -> (10.6066, 10.6066)
  line L10 (10.6066, 10.6066) -> (26.4632, -5.25)
  line L11 (24.9255, 17.5009) -> (37.1764, 5.25)
  line L12 (74.0694, 81.4941) -> (-3.7123, 3.7123)
  line L13 (10.6066, 10.6066) -> (6.8943, 14.3189)
  line L14 (24.9255, 17.5009) -> (14.3189, 6.8943)
  line L15 (6.8943, 14.3189) -> (17.5009, 24.9255)
  line L16 (17.5009, 24.9255) -> (24.9255, 17.5009)
  line L17 (24.9255, 17.5009) -> (2.1746, -5.25)
  line L18 (0, 7.4246) -> (7.4246, 0)
  point P0 (-2.2981, -2.2981)
  point P1 (24.9255, 17.5009)
  point P2 (17.5009, 24.9255)
  dimension "d29" = 30
  dimension "d30" = 45
  dimension "d31" = 10.5
  dimension "d32" = 6.5
  dimension "d38" = 15
  constraint coincident L0.start L1.start
  constraint horizontal L0
  constraint parallel L0 L1
  constraint tangent L2 A0
  constraint tangent A0 L3
  constraint parallel L2 L3
  constraint tangent L3 A1
  constraint tangent L2 A1
  constraint coincident L1.end A0.centre
  constraint parallel L1 L4
  constraint tangent L5 A2
  constraint tangent A2 L6
  constraint parallel L5 L6
  constraint tangent L6 A3
  constraint tangent L5 A3
  constraint parallel L4 L7
  constraint coincident L0.end A3.centre
  constraint concentric A1 A4
  constraint coincident A4 P0
  constraint perpendicular L8 L9
  constraint coincident L2 L10.end
  constraint perpendicular L9 L10
  constraint coincident P1 L11.start
  constraint coincident L3 L11.end
  constraint parallel L10 L11
  constraint coincident L12 L13.end
  constraint perpendicular L9 L13
  constraint coincident L10 L14.end
  constraint perpendicular L10 L14
  constraint coincident P2 L15.end
  constraint coincident L2 L17.end
  constraint perpendicular L11 L17
  constraint coincident L12 L18.start
  constraint coincident L17 L18.end
  constraint coincident L1 L18.end
  measures "d29" distance of L0.start L0.end
  measures "d30" distance of L0.start L1.end
  measures "d31" diameter of A0
  measures "d32" diameter of A2
  measures "d38" distance of L0.start L9.end
extrude "Extrude1'" add sketch "Sketch5" along normal blind 10 contours L2 A0 L3 L10 | L3 L8 L17 | L3 L10 L11 L14 L17 | L3 L10 L17 | L3 L8 L9 L10 L17 | L8 L9 L12 L13 | L10 L12 L13 L14 L15 L16 L17 bodies 2 in component "Cam version flap L = 30mm"
extrude "Extrude2'" add sketch "Sketch5" along normal blind 10 from surface at 169 contours L3 L8 L9 L17 L18 | L3 L9 L18 | L2 A0 L3 L10 | L3 L8 L9 | L3 L8 L9 L12 L18 | L3 L10 L11 L14 L17 | L3 L10 L17 | L3 L8 L9 L10 L17 | L8 L9 L12 L13 | L10 L12 L13 L14 L15 L16 L17 bodies 2 in component "Cam version flap L = 30mm"
component "Cam version flap L = 30mm" placed x (1, 0, 0) y (0, 1, 0) z (0, 0, 1) at (0, 0, 0)
equation "d5 = ( 10.5 / 2 ) * 1 mm"
equation "d10 = 110 mm - ( 10.5 / 2 ) * 1 mm"
equation "d16 = 180 mm - ( 10 * 2 ) * 1 mm"
equation "d19 = 29.75 mm - 10 mm"
equation "d20 = 89.5 mm - ( 5 * 2 ) * 1 mm"
equation "d23 = 80 mm - 10 mm"
equation "d35 = 170 mm - 1 mm"
